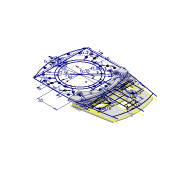
# Autodesk Inventor part: SensorHolder
Saved by Autodesk Inventor 2020.3 (Build 243373000, 373)
## iProperties
Created: 2021-06-20
Part Number: SensorHolder
Material: Generic
Document SubType Name: Modeling
Designer: Yusuf
Mass: 10.5667 g
Surface Area: 91.6742 cm^2
Volume: 10.5667 cm^3
Density: 1 g/cm^3
Appearance: Default
Author: Yusuf
Autodesk Inventor part; units mm, degrees
ref_plane "YZ Plane" through (0, 0, 0) normal (1, 0, 0) x (0, 1, 0)
ref_plane "XZ Plane" through (0, 0, 0) normal (0, 1, 0) x (-1, 0, 0)
ref_plane "XY Plane" through (0, 0, 0) normal (0, 0, 1) x (1, 0, 0)
sketch "Sketch1" plane through (0, 0, 0) normal (0, 1, 0) x (-1, 0, 0)
  line L0 (0, 0) -> (60, 0)
  line L1 (60, 0) -> (60, -81)
  line L2 (60, -81) -> (0, -81)
  line L3 (0, -81) -> (0, 0)
  line L4 (45, -21.6284) -> (15, -21.6284) construction
  line L5 (45, -81) -> (45, 0) construction
  line L6 (15, 0) -> (15, -81) construction
  circle A0 centre (40, -73.5) radius 1.5
  circle A1 centre (40, -7.5) radius 1.5
  circle A2 centre (20, -7.5) radius 1.5
  circle A3 centre (20, -73.5) radius 1.5
  line L7 (60, -40.5) -> (0, -40.5) construction
  line L8 (30, 0) -> (30, -81) construction
  circle A4 centre (30, -40.5) radius 24
  circle A5 centre (30, -40.5) radius 27.5
  circle A6 centre (57.1293, -36) radius 1.5
  circle A7 centre (57.1293, -45) radius 1.5
  circle A8 centre (25.5, -13.3707) radius 1.5
  circle A9 centre (34.5, -13.3707) radius 1.5
  circle A10 centre (2.8707, -45) radius 1.5
  circle A11 centre (2.8707, -36) radius 1.5
  circle A12 centre (34.5, -67.6293) radius 1.5
  circle A13 centre (25.5, -67.6293) radius 1.5
  circle A14 centre (30, -40.5) radius 40 construction
  arc A15 (60, -81) -> (60, 0) centre (-17.0125, -40.5) ccw
  circle A16 centre (30, -40.5) radius 36.28 construction
  circle A17 centre (65.9998, -36) radius 1.5
  circle A18 centre (65.9998, -45) radius 1.5
  circle A19 centre (-5.9998, -45) radius 1.5
  circle A20 centre (-5.9998, -36) radius 1.5
  arc A21 (0, 0) -> (0, -81) centre (77.0125, -40.5) ccw
  line L9 (30, -40.5) -> (-3.3536, -73.8536) construction
  circle A22 centre (1.7157, -68.7843) radius 1.5
  circle A23 centre (11.8404, -76.1403) radius 1.5
  circle A24 centre (23.7426, -80.0075) radius 1.5
  circle A25 centre (36.2574, -80.0075) radius 1.5
  circle A26 centre (48.1596, -76.1403) radius 1.5
  circle A27 centre (58.2843, -68.7843) radius 1.5
  circle A28 centre (65.6403, -58.6596) radius 1.5
  circle A29 centre (69.5075, -46.7574) radius 1.5
  circle A30 centre (69.5075, -34.2426) radius 1.5
  circle A31 centre (65.6403, -22.3404) radius 1.5
  circle A32 centre (58.2843, -12.2157) radius 1.5
  circle A33 centre (48.1596, -4.8597) radius 1.5
  circle A34 centre (36.2574, -0.9925) radius 1.5
  circle A35 centre (23.7426, -0.9925) radius 1.5
  circle A36 centre (11.8404, -4.8597) radius 1.5
  circle A37 centre (1.7157, -12.2157) radius 1.5
  circle A38 centre (-5.6403, -22.3404) radius 1.5
  circle A39 centre (-9.5075, -34.2426) radius 1.5
  circle A40 centre (-9.5075, -46.7574) radius 1.5
  circle A41 centre (-5.6403, -58.6596) radius 1.5
  circle A42 centre (48.1596, -68.7843) radius 1.5
  circle A43 centre (48.1596, -12.2157) radius 1.5
  circle A44 centre (11.8404, -12.2157) radius 1.5
  circle A45 centre (11.8404, -68.7843) radius 1.5
  line L10 (0, 0) -> (5, 0)
  arc A46 (5, 0) -> (6.3359, -13) centre (39.7267, -3) ccw
  arc A47 (6.3359, -13) -> (-5.0141, -31) centre (30, -40.5) ccw
  line L11 (-9.4798, -31) -> (7.9603, -31)
  line L12 (-10, -40.5) -> (70, -40.5) construction
  line L13 (-18.775, -8.5) -> (-32.775, -8.5)
  line L14 (-32.775, -8.5) -> (-32.775, -26.5)
  line L15 (-32.775, -26.5) -> (-18.775, -26.5)
  line L16 (-18.775, -26.5) -> (-18.775, -8.5)
  line L17 (-18.775, -54.5) -> (-37.775, -54.5)
  line L18 (-37.775, -54.5) -> (-37.775, -68.5)
  line L19 (-37.775, -68.5) -> (-18.775, -68.5)
  line L20 (-18.775, -68.5) -> (-18.775, -54.5)
  line L21 (-17.0125, -40.5) -> (-69.0232, -40.5)
  line L22 (-16.775, -6.5) -> (-23.775, -6.5)
  line L23 (-23.775, -6.5) -> (-23.775, -28.5)
  line L24 (-23.775, -28.5) -> (-16.775, -28.5)
  line L25 (-16.775, -28.5) -> (-16.775, -6.5)
  line L26 (-16.775, -52.5) -> (-23.775, -52.5)
  line L27 (-23.775, -52.5) -> (-23.775, -70.5)
  line L28 (-23.775, -70.5) -> (-16.775, -70.5)
  line L29 (-16.775, -70.5) -> (-16.775, -52.5)
  circle A48 centre (-30.7674, -10.5) radius 1.25
  circle A49 centre (-30.7674, -24.5) radius 1.25
  circle A50 centre (-35.775, -56.5) radius 1.25
  line L30 (-16.775, -32.5) -> (-49.775, -32.5)
  line L31 (-51.775, -34.5) -> (-51.775, -46.5)
  line L32 (-49.775, -48.5) -> (-16.775, -48.5)
  line L33 (-16.775, -48.5) -> (-16.775, -32.5)
  line L34 (-16.775, -43.5) -> (-38.775, -43.5) construction
  line L35 (-32.0174, -32.5) -> (-46.0174, -32.5)
  line L36 (-46.0174, -32.5) -> (-46.0174, -48.5)
  line L37 (-46.0174, -48.5) -> (-32.0174, -48.5)
  line L38 (-32.0174, -48.5) -> (-32.0174, -32.5)
  line L39 (0, 0) -> (-59.1614, -10.4318)
  line L40 (0, -81) -> (-59.1614, -70.5682)
  arc A51 (-51.775, -9.1293) -> (-51.775, -71.8707) centre (29.3856, -40.5) ccw
  arc A52 (-49.775, -32.5) -> (-51.775, -34.5) centre (-49.775, -34.5) ccw
  arc A53 (-51.775, -46.5) -> (-49.775, -48.5) centre (-49.775, -46.5) ccw
  arc A54 (6.3359, -68) -> (5, -81) centre (39.7267, -78) ccw
  arc A55 (-5.0141, -50) -> (6.3359, -68) centre (30, -40.5) ccw
  line L41 (-9.4798, -50) -> (7.9603, -50)
  arc A56 (-4.4033, -0.7764) -> (-4.4033, -80.2236) centre (73.0125, -40.5) ccw
  circle A57 centre (1.7157, -12.2157) radius 3.25
  circle A58 centre (1.7157, -68.7843) radius 3.25
  arc A59 (6.3359, -13) -> (7.176, -15.4657) centre (39.7267, -3) ccw
  arc A60 (7.176, -15.4657) -> (0, -20.0981) centre (14.726, -35.0357) ccw
  arc A61 (7.176, -65.5343) -> (6.3359, -68) centre (39.7267, -78) ccw
  arc A62 (0, -60.9019) -> (7.176, -65.5343) centre (14.726, -45.9643) ccw
  point P0 (30, -21.6284)
  point P1 (-18.775, -17.5)
  point P2 (-18.775, -61.5)
  point P3 (-51.775, -48.5)
  point P4 (-51.775, -32.5)
  point P5 (-16.775, -40.5)
  point P6 (-16.775, -61.5)
  point P7 (-51.775, -40.5)
  point P8 (-14, -40.5)
  point P9 (5, -81)
  point P10 (0, -60.9019)
  dimension "d18" = 48
  dimension "d6" = 60
  dimension "d7" = 81
  dimension "d8" = 3
  dimension "d9" = 7.5
  dimension "d10" = 5
  dimension "d11" = 30
  dimension "d12" = 3
  dimension "d13" = 7.5
  dimension "d14" = 5
  dimension "d15" = 3
  dimension "d16" = 3
  dimension "d17" = 5
  dimension "d19" = 55
  dimension "d20" = 3
  dimension "d21" = 4.5
  dimension "d22" = 3
  dimension "d23" = 4.5
  dimension "d24" = 360
  dimension "d25" = 80
  dimension "d26" = 72.56
  dimension "d27" = 3
  dimension "d28" = 3
  dimension "d29" = 360
  dimension "d30" = 45
  dimension "d31" = 3
  dimension "d32" = 360
  dimension "d33" = 3
  dimension "d34" = 3
  dimension "d35" = 3
  dimension "d36" = 3
  dimension "d37" = 5
  dimension "d38" = 5
  dimension "d39" = 30
  dimension "d40" = 40.5
  dimension "d41" = 14
  dimension "d42" = 18
  dimension "d43" = 19
  dimension "d44" = 14
  dimension "d45" = 7
  dimension "d46" = 2
  dimension "d47" = 2
  dimension "d48" = 2
  dimension "d49" = 2
  dimension "d50" = 2
  dimension "d51" = 2
  dimension "d52" = 7
  dimension "d53" = 2.5
  dimension "d54" = 2.5
  dimension "d55" = 2
  dimension "d56" = 2
  dimension "d57" = 2.5
  dimension "d58" = 2
  dimension "d59" = 2
  dimension "d60" = 35
  dimension "d61" = 16
  dimension "d62" = 4
  dimension "d63" = 4
  dimension "d64" = 22
  dimension "d65" = 14
  dimension "d66" = 80
  dimension "d67" = 80
  dimension "d68" = 2
  dimension "d69" = 4
  dimension "d78" = 6.5
  constraints: 84 end point, 62 centre point, 43 point on circle, 23 point on line, 14 parallel, 12 midpoint, 11 symmetric about line, 10 horizontal, 10 horizontal alignment, 9 perpendicular, 9 vertical alignment, 6 coincident, 5 equal radius, 5 tangent, 75 other
  measures "d6" distance of L2.start L2.end
  measures "d7" distance of L0.end L2.start
  measures "d8" diameter of A0
  measures "d9" distance from line of A0.centre L2
  measures "d10" distance from line of L5 A0.centre
  measures "d11" distance between parallel lines of L6 L5
  measures "d12" diameter of A1
  measures "d13" distance from line of L0 A1.centre
  measures "d14" distance from line of L5 A1.centre
  measures "d15" diameter of A2
  measures "d16" diameter of A3
  measures "d17" distance from line of L6 A2.centre
  measures "d19" diameter of A5
  measures "d20" diameter of A6
  measures "d21" distance from line of A6.centre L7
  measures "d22" diameter of A7
  measures "d23" distance from line of L7 A7.centre
  measures "d25" diameter of A14
  measures "d26" diameter of A16
  measures "d27" diameter of A17
  measures "d28" diameter of A18
  measures "d30" angle of L8 L9
  measures "d31" diameter of A22
  measures "d33" diameter of A42
  measures "d34" diameter of A43
  measures "d35" diameter of A44
  measures "d36" diameter of A45
  measures "d37" distance of L0.start L10.end
  measures "d38" distance from line of A20.centre L11
  measures "d39" horizontal distance of point (0, 0) point (30, -40.5)
  measures "d40" vertical distance of point (0, 0) point (30, -40.5)
  measures "d41" distance of L15.end L14.end
  measures "d42" distance of L14.end L13.end
  measures "d43" distance of L19.end L18.end
  measures "d44" distance of L18.end L17.end
  measures "d45" distance of L24.end L23.end
  measures "d46" distance between parallel lines of L16 L25
  measures "d47" distance between parallel lines of L15 L24
  measures "d48" distance between parallel lines of L13 L22
  measures "d49" distance between parallel lines of L29 L20
  measures "d50" distance between parallel lines of L26 L17
  measures "d51" distance between parallel lines of L28 L19
  measures "d52" distance between parallel lines of L27 L29
  measures "d53" diameter of A48
  measures "d54" diameter of A49
  measures "d55" distance from line of L13 A48.centre
  measures "d56" distance from line of L15 A49.centre
  measures "d57" diameter of A50
  measures "d58" distance from line of L17 A50.centre
  measures "d59" distance from line of L18 A50.centre
  measures "d60" distance of L32.end point (-51.775, -48.5)
  measures "d61" distance of point (-51.775, -32.5) point (-51.775, -48.5)
  measures "d62" distance between parallel lines of L26 L32
  measures "d63" distance between parallel lines of L30 L24
  measures "d64" distance of L34.start L34.end
  measures "d65" distance of L37.end L36.end
  measures "d66" angle of L3 L39
  measures "d67" angle of L3 L40
  measures "d68" radius of A52
  measures "d69" distance of L12.start point (-14, -40.5)
  measures "d78" diameter of A57
extrude "Extrusion1" add sketch "Sketch1" along normal blind 2 contours L0 A46 A47 L3 A57 | L3 A57 A47 L11 A21 | A21 A39 A40 L40 A56 L39 | A59 A60 A47 | A21 A39 | L3 A58 A55 A54 L2 | A21 L41 A55 L3 A58 | A21 A40 | A62 A61 A55 picked at (-10.1825, -34.1938) picked at (-10.1825, -46.8062)
extrude "Extrusion2" add sketch "Sketch1" against normal blind 4 contours A21 A39 A40 L40 A56 L39 | A21 A39 | A21 A40 picked at (-10.1825, -34.1938) picked at (-10.1825, -46.8062)
ref_plane "Work Plane1" through (0, -5.5, 0) normal (0, -1, 0) x (1, 0, 0)
sketch "Sketch2" plane through (0, -5.5, 0) normal (0, -1, 0) x (1, 0, 0)
  line L0 (0, -81) -> (59.1614, -70.5682) projected
  arc A0 (51.775, -71.8707) -> (51.775, -9.1293) centre (-29.3856, -40.5) ccw projected
  line L1 (49.775, -48.5) -> (16.775, -48.5) projected
  arc A1 (49.775, -48.5) -> (51.775, -46.5) centre (49.775, -46.5) ccw projected
  line L2 (51.775, -34.5) -> (51.775, -46.5) projected
  arc A2 (51.775, -34.5) -> (49.775, -32.5) centre (49.775, -34.5) ccw projected
  line L3 (16.775, -32.5) -> (49.775, -32.5) projected
  line L4 (46.0174, -32.5) -> (46.0174, -48.5) projected
  line L5 (32.0174, -48.5) -> (32.0174, -32.5) projected
  line L6 (16.775, -48.5) -> (16.775, -32.5) projected
  arc A3 (4.4033, -80.2236) -> (4.4033, -0.7764) centre (-73.0125, -40.5) ccw projected
  arc A4 (0, -81) -> (0, 0) centre (-77.0125, -40.5) ccw projected
  line L7 (37.775, -68.5) -> (18.775, -68.5) projected
  line L8 (37.775, -54.5) -> (37.775, -68.5) projected
  line L9 (18.775, -54.5) -> (37.775, -54.5) projected
  circle A5 centre (35.775, -56.5) radius 1.25 projected
  line L10 (23.775, -52.5) -> (23.775, -70.5) projected
  line L11 (23.775, -70.5) -> (16.775, -70.5) projected
  line L12 (16.775, -70.5) -> (16.775, -52.5) projected
  line L13 (18.775, -68.5) -> (18.775, -54.5) projected
  line L14 (16.775, -52.5) -> (23.775, -52.5) projected
  line L15 (32.775, -26.5) -> (18.775, -26.5) projected
  circle A6 centre (30.7674, -24.5) radius 1.25 projected
  line L16 (32.775, -8.5) -> (32.775, -26.5) projected
  circle A7 centre (30.7674, -10.5) radius 1.25 projected
  line L17 (18.775, -8.5) -> (32.775, -8.5) projected
  line L18 (0, 0) -> (59.1614, -10.4318) projected
  line L19 (23.775, -6.5) -> (23.775, -28.5) projected
  line L20 (16.775, -6.5) -> (23.775, -6.5) projected
  line L21 (16.775, -28.5) -> (16.775, -6.5) projected
  line L22 (18.775, -26.5) -> (18.775, -8.5) projected
  line L23 (23.775, -28.5) -> (16.775, -28.5) projected
  line L24 (17.0125, -40.5) -> (69.0232, -40.5) projected
  point P0 (23.775, -26.5)
  point P1 (23.775, -8.5)
  point P2 (23.775, -68.5)
  point P3 (23.775, -54.5)
extrude "Extrusion3" add sketch "Sketch2" along normal blind 2.5 contours A4 L18 A3 L0 | A3 L18 A0 L0 | L1 L4 L24 L2 A1 | L1 L6 L3 L5 | L4 L3 A2 L2 L24 | L7 L10 L9 L8 | L15 L19 L17 L16
extrude "Extrusion4" add sketch "Sketch2" against normal up to surface (1.5 mm away) contours A4 L18 A3 L0
fillet "Fillet1" radius 2 3 edges at (46.0174, -6.75, -32.5) (46.0174, -6.75, -48.5) (14, -5.5, -40.5)
equation "\"d11\" = 0.5 * d6"
equation "\"d12\" = d8"
equation "\"d15\" = d8"
equation "\"d16\" = d8"
equation "\"d22\" = d8"
equation "\"d27\" = d8"
equation "\"d28\" = d8"
equation "\"d31\" = d8"
equation "\"d33\" = d8"
equation "\"d34\" = d8"
equation "\"d35\" = d8"
equation "\"d36\" = d8"
body "Solid1"
